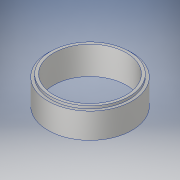
# Autodesk Inventor part: aluminum_retainer
Saved by Autodesk Inventor 2017 SP1 (Build 210196100, 196)
## iProperties
Created: 2016-07-25
Part Number: aluminum_retainer
Material: Aluminum 6061
Document SubType Name: Modeling
Designer: Jared
Density: 2.7 g/cm^3
Appearance: Aluminum - Flat
Author: Jared
Autodesk Inventor part; units mm, degrees
ref_plane "YZ Plane" through (0, 0, 0) normal (1, 0, 0) x (0, 1, 0)
ref_plane "XZ Plane" through (0, 0, 0) normal (0, 1, 0) x (-1, 0, 0)
ref_plane "XY Plane" through (0, 0, 0) normal (0, 0, 1) x (1, 0, 0)
sketch "Sketch1" plane through (0, 0, 0) normal (0, 0, 1) x (1, 0, 0)
  line L0 (0, 25.4) -> (-28.702, 25.4) construction
  line L1 (0, 25.4) -> (-95.25, 25.4) construction
  line L2 (-95.25, 25.4) -> (-92.075, 25.4) construction
  line L3 (-92.075, 25.4) -> (-84.455, 21.8467) construction
  line L4 (-92.075, 25.4) -> (-92.075, 22.4389) construction
  line L5 (-92.075, 0) -> (-95.25, 0)
  line L6 (-28.702, 59.0535) -> (-28.702, -92.5226) construction
  arc A0 (-28.9184, -9.8402) -> (-32.3684, -2.4417) centre (-35.052, -8.1967) ccw
  line L7 (-76.2, -186.2977) -> (-28.702, -9.0327)
  line L8 (-92.075, 25.4) -> (-92.075, 0)
  line L9 (-92.075, 25.4) -> (-32.3684, -2.4417)
  line L10 (-28.702, -8.1967) -> (-60.452, -8.1967) construction
  line L11 (-60.452, -127.5253) -> (-54.102, -127.5253) construction
  line L12 (-54.102, -127.5253) -> (-54.102, -103.8268) construction
  line L13 (-54.102, -103.8268) -> (-60.452, -103.8268)
  line L14 (-60.452, 10.654) -> (-60.452, 1.129) construction
  line L15 (-60.452, 10.654) -> (-60.452, 4.1232) construction
  line L16 (-60.452, 4.1232) -> (-46.4468, 4.1232)
  line L17 (-95.25, 0) -> (-95.25, -12.7) construction
  line L18 (-60.452, -12.7) -> (-73.152, -12.7) construction
  line L19 (-95.25, -12.7) -> (-95.25, -25.4) construction
  line L20 (-95.25, -25.4) -> (-95.25, -88.9) construction
  line L21 (-95.25, -88.9) -> (-82.55, -88.9) construction
  line L22 (-82.55, -88.9) -> (-82.55, -25.4) construction
  line L23 (-95.25, -25.4) -> (-82.55, -25.4)
  line L24 (-82.55, -25.4) -> (-82.55, -88.9)
  line L25 (-82.55, -88.9) -> (-95.25, -88.9)
  line L26 (-95.25, -12.7) -> (-73.152, -12.7)
  line L27 (-73.152, -139.3746) -> (-63.627, -139.3746)
  line L28 (-82.55, -88.9) -> (-82.55, -186.2977)
  line L29 (-82.55, -186.2977) -> (-76.2, -186.2977)
  line L30 (-73.152, -12.7) -> (-73.152, -139.3746)
  line L31 (-88.9, -25.4) -> (-88.9, -31.3436)
  line L32 (-88.9, -31.3436) -> (-95.25, -31.3436)
  line L33 (-95.25, 0) -> (-95.25, -25.4)
  line L34 (-95.25, -31.3436) -> (-95.25, -88.9)
  line L35 (-88.9, -160.8977) -> (-88.9, -221.8454)
  line L36 (-28.9184, -9.8402) -> (-85.725, -221.8454)
  line L37 (-85.725, -221.8454) -> (-88.9, -221.8454)
  line L38 (-82.55, -160.8977) -> (-88.9, -160.8977)
  line L39 (-66.802, -38.1) -> (-66.802, 4.1232)
  line L40 (-66.802, 4.1232) -> (-60.452, 4.1232)
  line L41 (-66.802, -38.1) -> (-60.452, -103.8268)
  line L42 (-60.452, 10.654) -> (-60.452, 4.1232) construction
  line L43 (-60.452, -8.1967) -> (-60.452, -12.7) construction
  line L44 (-60.452, -103.8268) -> (-60.452, -127.5253) construction
  line L45 (0, 59.6457) -> (0, -91.9304) construction
  line L46 (-73.152, -38.1) -> (-69.977, -38.1)
  line L47 (-69.977, -38.1) -> (-69.977, -12.7)
  line L48 (-66.802, -12.7) -> (-69.977, -12.7)
  point P0 (0, 0)
  point P1 (-95.25, -256.5049)
  point P2 (-88.7095, 22.4389)
  dimension "d0" = 28.702
  dimension "d1" = 95.25
  dimension "d2" = 3.175
  dimension "d3" = 25
  dimension "d5" = 25.4
  dimension "d6" = 25.4
  dimension "d8" = 12.7
  dimension "d12" = 31.75
  dimension "d13" = 6.35
  dimension "d16" = 12.7
  dimension "d17" = 12.7
  dimension "d18" = 12.7
  dimension "d19" = 63.5
  dimension "d20" = 12.7
  dimension "d22" = 9.525
  dimension "d23" = 6.35
  dimension "d25" = 5.9436
  dimension "d27" = 3.175
  dimension "d28" = 6.35
  dimension "d29" = 25.4
  dimension "d30" = 107.95
  dimension "d31" = 6.35
  dimension "d33" = 20.3552
  dimension "d34" = 15
  dimension "d35" = 3.175
  dimension "d36" = 25.4
  constraints: 98 end point, 26 perpendicular, 20 point on line, 16 vertical, 5 tangent, 5 vertical alignment, 4 horizontal, 3 midpoint, 3 point on circle, 2 collinear, 1 centre point, 1 horizontal alignment
  measures "d0" distance of L0.start L0.end
  measures "d1" distance of L0.start L1.end
  measures "d2" distance of L2.end L1.end
  measures "d3" angle of L1 L3
  measures "d5" distance of point (0, 0) L0.start
  measures "d6" distance of L2.end L5.start
  measures "d8" diameter of A0
  measures "d12" distance of L10.end L10.start
  measures "d13" distance of L11.start L11.end
  measures "d16" distance of L5.end L17.end
  measures "d17" distance of L18.start L18.end
  measures "d18" distance of L17.end L19.end
  measures "d19" distance of L20.end L19.end
  measures "d20" distance of L20.end L21.end
  measures "d22" distance of L27.start L27.end
  measures "d23" distance of L28.end L7.start
  measures "d25" distance of L31.start L31.end
  measures "d27" distance of L35.end L36.end
  measures "d28" distance of L38.start L35.start
  measures "d29" distance from line of L28.end L38
  measures "d30" distance of L13.end L15.end
  measures "d31" distance between parallel lines of L30 L39
  measures "d33" distance of L16.end L39.end
  measures "d34" angle of L6 L36
  measures "d35" distance of L48.start L47.end
  measures "d36" distance from line of L18.end L46
revolve "Revolution1" add sketch "Sketch1" angle 360 about axis through (0, 59.6457, 0) along (0, -1, 0) contours L23 L24 L25 L34 L32 L31
body "Solid1"
